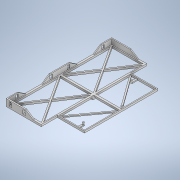
# Autodesk Inventor part: Wexterås-Hållare v2
Saved by Autodesk Inventor 2021 (Build 250183000, 183)
## iProperties
Created: 2024-12-11
Part Number: Wexterås-Hållare v2
Material: Generic
Document SubType Name: Modeling
Designer: 24ludrum
Density: 1 g/cm^3
Appearance: Default
Author: 24ludrum
Autodesk Inventor part; units mm, degrees
ref_plane "YZ Plane" through (0, 0, 0) normal (1, 0, 0) x (0, 1, 0)
ref_plane "XZ Plane" through (0, 0, 0) normal (0, 1, 0) x (-1, 0, 0)
ref_plane "XY Plane" through (0, 0, 0) normal (0, 0, 1) x (1, 0, 0)
sketch "Sketch1" plane through (0, 0, 0) normal (0, 1, 0) x (-1, 0, 0)
  line L0 (54, 0) -> (55.5, 0)
  line L1 (55.5, 0) -> (55.5, 82)
  line L2 (55.5, 82) -> (55.5, 83.5)
  line L3 (55.5, 83.5) -> (54, 83.5)
  line L4 (0, 83.5) -> (0, 82)
  line L5 (54, 82) -> (54, 80.5)
  line L6 (54, 82) -> (52.5, 82)
  line L7 (54, 0) -> (54, 1.5)
  line L8 (54, 1.5) -> (54, 80.5)
  line L9 (54, 0) -> (52.5, 0)
  line L10 (0, 1.5) -> (0, 0)
  line L11 (0, 0) -> (1.5, 0)
  line L12 (52.5, 82) -> (0, 1.5)
  line L13 (1.5, 0) -> (54, 80.5)
  line L14 (0, 83.5) -> (1.5, 83.5)
  line L15 (54, 83.5) -> (0, 83.5)
  line L16 (0, 82) -> (1.5, 82)
  line L17 (0, 82) -> (0, 80.5)
  line L18 (52.5, 82) -> (1.5, 82)
  line L19 (52.5, 0) -> (0, 80.5)
  line L20 (1.5, 82) -> (54, 1.5)
  line L21 (0, 0) -> (0, -0.1)
  line L22 (54, 0) -> (54, -0.1)
  line L23 (0, 0) -> (-43.1, 0)
  line L24 (0, 58) -> (0, 56.5)
  line L25 (0, 56.5) -> (0, 1.5)
  line L26 (-43.1, 1.5) -> (-43.1, 0)
  line L27 (-43.1, 58) -> (-43.1, 56.5)
  line L28 (-43.1, 56.5) -> (-43.1, 1.5)
  line L29 (0, 80.5) -> (0, 58)
  line L30 (1.5, 1.5) -> (52.5, 1.5)
  line L31 (52.5, 1.5) -> (52.5, 80.5)
  line L32 (0, 58) -> (-1.5, 58)
  line L33 (-43.1, 58) -> (-41.6, 58)
  line L34 (-1.5, 58) -> (-41.6, 58)
  line L35 (-41.6, 1.4999) -> (-1.3749, 1.4999)
  line L36 (-41.6, 1.4999) -> (-41.6, 56.5001)
  line L37 (52.5, 0) -> (1.5, 0)
  line L38 (55.5, 0) -> (55.5, -0.1)
  line L39 (52.5, 80.5) -> (1.5, 80.5)
  line L40 (1.5, 80.5) -> (1.5, 1.5)
  line L41 (-1.3749, 56.5001) -> (-41.6, 56.5001)
  line L42 (-1.3749, 56.5001) -> (-1.3749, 1.4999)
  line L43 (54, -0.1) -> (0, -0.1)
  line L44 (0, -0.1) -> (-43.1, -0.1)
  line L45 (-43.1, -0.1) -> (-43.1, 0)
  line L46 (54, -0.1) -> (55.5, -0.1)
  point P0 (27, 39.1)
  point P1 (51.5217, 1.5)
  point P2 (2.4783, 1.5)
  point P3 (25.7609, 41)
  point P4 (1.5, 3.8)
  point P5 (1.5, 78.2)
  point P6 (28.2391, 41)
  point P7 (52.5, 78.2)
  point P8 (52.5, 3.8)
  point P9 (27, 42.9)
  point P10 (2.4783, 80.5)
  point P11 (51.5217, 80.5)
  dimension "d0" = 82
  dimension "d1" = 54
  dimension "d2" = 82
  dimension "d3" = 1.5
  dimension "d4" = 1.5
  dimension "d5" = 1.5
  dimension "d6" = 1.5
  dimension "d8" = 1.5
  dimension "d9" = 1.5
  dimension "d10" = 1.5
  dimension "d12" = 1.5
  dimension "d13" = 1.5
  dimension "d14" = 1.5
  dimension "d15" = 1.5
  dimension "d16" = 1.5
  dimension "d17" = 0.1
  dimension "d18" = 0.1
  dimension "d19" = 43.1
  dimension "d20" = 58
  dimension "d21" = 1.5
  dimension "d22" = 1.5
  dimension "d23" = 55
  dimension "d24" = 1.5
  dimension "d25" = 1.5
  dimension "d26" = 51
  dimension "d27" = 54
  dimension "d28" = 51
  dimension "d31" = 40.2251
  dimension "d33" = 55.0001
  dimension "d34" = 1.5
  dimension "d35" = 0.1
  dimension "d37" = 1.5
  dimension "d38" = 1.4999
  dimension "d39" = 1.5
  constraints: 94 end point, 13 horizontal, 13 vertical, 9 perpendicular, 3 parallel, 2 point on line, 1 collinear
  measures "d0" distance of L0.start L5.start
  measures "d1" distance of L5.start L4.end
  measures "d2" distance of L0.end L1.end
  measures "d3" distance of L0.start L0.end
  measures "d4" distance of L1.end L2.end
  measures "d5" distance of L5.start L5.end
  measures "d6" distance of L5.start L6.end
  measures "d8" distance of L0.start L7.end
  measures "d9" distance of L0.start L9.end
  measures "d10" distance of L4.start L4.end
  measures "d12" distance of L10.end L11.end
  measures "d13" distance of L10.start L10.end
  measures "d14" distance of L4.start L14.end
  measures "d15" distance of L4.end L17.end
  measures "d16" distance of L4.end L16.end
  measures "d17" distance of L10.end L21.end
  measures "d18" distance of L0.start L22.end
  measures "d19" distance of L10.end L23.end
  measures "d20" distance of L23.end L27.start
  measures "d21" distance of L24.start L24.end
  measures "d22" distance of L27.start L27.end
  measures "d23" distance of L27.end L26.start
  measures "d24" distance of L24.start L32.end
  measures "d25" distance of L27.start L33.end
  measures "d26" distance of L30.start L30.end
  measures "d27" distance of L3.end L4.start
  measures "d28" distance of L18.start L16.end
  measures "d31" distance of L35.start L35.end
  measures "d33" distance of L35.start L36.end
  measures "d34" distance between parallel lines of L8 L31
  measures "d35" distance of L0.end L38.end
  measures "d37" distance between parallel lines of L39 L18
  measures "d38" distance between parallel lines of L34 L41
  measures "d39" distance between parallel lines of L28 L36
extrude "Extrusion1" add sketch "Sketch1" along normal blind 3 contours L7 L8 L5 L6 L18 L16 L4 L14 L15 L3 L2 L1 L0 | L9 L19 L30 L31 L20 L7 | L22 L43 L21 L11 L37 L9 | L20 L31 L13 L8 | L37 L13 L30 L19 | L13 L31 L39 L12 L6 L5 | L31 L30 L19 L13 L20 | L11 L10 L12 L40 L30 L13 | L44 L45 L23 L21 | L13 L20 L12 L39 L31 | L13 L19 L12 L20 | L13 L30 L40 L12 L19 | L23 L26 L28 L27 L33 L34 L32 L24 L25 L10 | L12 L39 L20 L18 | L12 L19 L40 L39 L20 | L25 L24 L29 L19 L40 L12 | L20 L39 L40 L19 L17 L16
sketch "Sketch3" plane through (-55.5, 0, 0) normal (-1, 0, 0) x (0, 0, 1)
  line L0 (3.8, 3) -> (78.2, 3) projected
  line L1 (11.2989, 4) -> (11.2989, 11)
  line L2 (11.2989, 4) -> (15.4989, 4)
  line L3 (15.4989, 11) -> (11.2989, 11)
  line L4 (15.4989, 11) -> (15.4989, 9.2)
  line L5 (15.4989, 9.2) -> (15.4989, 4)
  line L6 (15.4989, 9.2) -> (11.2989, 9.2)
  line L7 (58, 3) -> (0, 3) projected
  line L8 (11.2989, 11) -> (-0.7359, 2.9768)
  line L9 (15.4989, 11) -> (27.5338, 2.9768)
  line L10 (0, 3) -> (40.25, 3) construction
  line L11 (40.25, 3) -> (40.25, 23.325) construction
  line L12 (27.5338, 2.9768) -> (-0.7359, 2.9768)
  line L13 (70, 4) -> (70, 11)
  line L14 (70, 4) -> (65.8, 4)
  line L15 (65.8, 11) -> (70, 11)
  line L16 (65.8, 11) -> (65.8, 9.2)
  line L17 (65.8, 9.2) -> (65.8, 4)
  line L18 (65.8, 9.2) -> (70, 9.2)
  line L19 (65.8, 11) -> (53.8, 3)
  line L20 (56.5001, 0) -> (56.5001, 3) projected
  line L21 (83.5, 3) -> (58, 3) projected
  line L22 (56.5001, 3) -> (83.5, 3)
  line L23 (83.5, 3) -> (83.5, 11)
  line L24 (83.5, 11) -> (70, 11)
  line L25 (58, 3) -> (-0.1, 3) projected
  line L26 (55.3, 3) -> (58, 3)
  line L27 (55.3, 3) -> (83.5, 3)
  line L28 (53.8, 3) -> (55.3, 3)
  line L29 (0, 3) -> (-0.1, 3)
  line L30 (-0.1, 3) -> (0, 3) construction
  line L31 (-0.1, 3) -> (0, 3) construction
  line L32 (0, 3) -> (-0.1, 3) construction
  line L33 (83.5, 4) -> (15.5, 4) construction
  point P0 (0, 0)
  point P1 (80.5, 3)
  point P2 (53.8, 3)
  point P3 (27.4989, 3)
  point P4 (70, 11)
  point P5 (0, 3)
  point P6 (27.4989, 3)
  dimension "d45" = 4.2
  dimension "d47" = 5.2
  dimension "d49" = 1
  dimension "d50" = 7
  dimension "d52" = 33.69
  dimension "d55" = 1.8
  dimension "d56" = 33.69
  dimension "d57" = 40.25
  dimension "d93" = 8
  dimension "d94" = 13.5
  dimension "d95" = 33.69
  dimension "d96" = 4.2
  dimension "d97" = 4.2
  dimension "d98" = 1.8
  dimension "d99" = 12
  dimension "d100" = 5.2
  dimension "d101" = 7
  dimension "d102" = 4.2
  dimension "d103" = 1
  dimension "d104" = 90
  dimension "d112" = 68
  constraints: 56 end point, 7 horizontal, 4 point on line, 4 vertical, 1 parallel, 1 perpendicular, 1 symmetric about line, 1 other
  measures "d45" distance of L1.start L2.end
  measures "d47" distance of L4.end L2.end
  measures "d49" distance between parallel lines of L0 L2
  measures "d50" distance of L1.start L1.end
  measures "d52" angle of L7 L8
  measures "d55" distance between parallel lines of L6 L3
  measures "d56" angle of L0 L9
  measures "d57" distance of L7.end L10.end
  measures "d93" distance of L21.start L23.end
  measures "d94" distance of L23.end L24.end
  measures "d95" angle of L0 L19
  measures "d96" distance of L13.start L14.end
  measures "d97" distance of L18.start L18.end
  measures "d98" distance between parallel lines of L18 L15
  measures "d99" horizontal distance of L16.start L19.end
  measures "d100" distance of L18.start L14.end
  measures "d101" distance of L13.start L13.end
  measures "d102" distance of L16.start L13.end
  measures "d103" distance between parallel lines of L21 L14
  measures "d104" angle of L24 L13
  measures "d112" distance of L33.start L33.end
extrude "Extrusion2" add sketch "Sketch3" against normal blind 1.5 contours L19 L16 L17 L14 L13 L24 L23 L21 L0 | L15 L13 L18 L16 | L2 L5 L4 L9 L12 L8 L1 | L1 L3 L4 L6
extrude "Extrusion3" add sketch "Sketch1" along normal blind 3 contours L0 L38 L46 L22
mirror "Mirror1" about plane through (43.1, 0, -0.1) normal (0, 0, -1) of "Extrusion1", "Extrusion2"
sketch "Sketch4" plane through (-55.5, 0, 83.5) normal (0, 0, 1) x (1, 0, 0)
  line L0 (1.5, 0) -> (0, 0) projected
  line L1 (0, 0) -> (0, 11) projected
  line L2 (0, 0) -> (0, 11)
  line L3 (0, 11) -> (1.5, 11) projected
  line L4 (0, 11) -> (1.5, 11)
  line L5 (1.5, 11) -> (4.55, 11)
  line L6 (4.55, 11) -> (4.55, 4.6854)
  line L7 (4.55, 4.6854) -> (4.55, 0)
  line L8 (3.9783, 3) -> (53.0217, 3) projected
  line L9 (4.55, 3) -> (0, 3)
  line L10 (1.5, 3.4007) -> (1.5, 11) projected
  line L11 (1.5, 11) -> (1.5, 3)
  line L12 (4.55, 9) -> (8.75, 9)
  line L13 (4.55, 11) -> (8.75, 11)
  line L14 (8.75, 11) -> (8.75, 3)
  line L15 (8.75, 11) -> (26.55, 11)
  line L16 (26.55, 11) -> (26.55, 3)
  line L17 (26.55, 11) -> (30.75, 11)
  line L18 (26.55, 9) -> (32.35, 9)
  line L19 (30.75, 11) -> (30.75, 3)
  line L20 (30.75, 11) -> (43.0689, 3)
  line L21 (53.0217, 3) -> (3.9783, 3) projected
  point P0 (55.5, 0)
  point P1 (30.75, 9)
  dimension "d62" = 3.05
  dimension "d64" = 4.2
  dimension "d65" = 2
  dimension "d66" = 4.2
  dimension "d67" = 17.8
  dimension "d68" = 4.2
  dimension "d69" = 2
  dimension "d70" = 33
  constraints: 32 end point, 10 point on line, 5 horizontal, 4 perpendicular, 3 collinear, 2 vertical
  measures "d62" distance of L3.end L5.end
  measures "d64" distance of L12.start L12.end
  measures "d65" distance between parallel lines of L12 L13
  measures "d66" distance of L5.end L13.end
  measures "d67" distance of L13.end L15.end
  measures "d68" distance of L15.end L17.end
  measures "d69" distance between parallel lines of L18 L17
  measures "d70" angle of L20 L8
extrude "Extrusion4" add sketch "Sketch4" against normal blind 2 contours L11 L10 L5 L6 L7 L8 L9 | L13 L14 L12 L6 | L15 L16 L8 L14 | L17 L19 L18 L16 | L20 L8 L19
sketch "Sketch5" plane through (0, 0, -83.7) normal (0, 0, -1) x (-1, 0, 0)
  line L0 (55.5, 11) -> (54, 11) projected
  line L1 (54, 11) -> (24.75, 11) projected
  line L2 (55.5, 11) -> (24.75, 11)
  line L3 (24.75, 11) -> (12.4311, 3) projected
  line L4 (24.75, 11) -> (12.4311, 3)
  line L5 (12.4311, 3) -> (55.5, 3)
  line L6 (55.5, 3) -> (55.5, 11)
  point P0 (0, 0)
  constraints: 8 end point, 1 collinear, 1 horizontal, 1 parallel, 1 perpendicular
extrude "Extrusion5" add sketch "Sketch5" against normal blind 1.5
sketch "Sketch6" plane through (0, 0, 0) normal (0, -1, 0) x (1, 0, 0)
  line L0 (1.3749, 56.5001) -> (1.3749, 1.4999) construction
  line L1 (1.3749, 1.4999) -> (3.3749, 1.4999) construction
  line L2 (1.3749, 1.4999) -> (41.6, 1.4999) construction
  line L3 (1.3749, 1.4999) -> (1.3749, 4.4999) construction
  line L4 (1.3749, 4.4999) -> (3.3749, 4.4999) construction
  circle A0 centre (3.3749, 4.4999) radius 1.4 construction
  line L5 (3.3749, 5.8999) -> (1.3749, 5.8999) construction
  line L6 (3.3749, 3.0999) -> (3.3749, 1.4999) construction
  line L7 (3.3749, 3.0999) -> (3.3749, 1.4999)
  line L8 (3.3749, 5.8999) -> (1.3749, 5.8999)
  line L9 (1.3749, 5.8999) -> (1.3749, 1.4999)
  line L10 (3.3749, 1.4999) -> (1.3749, 1.4999)
  circle A1 centre (3.3749, 4.4999) radius 1.4
  line L11 (3.3749, 4.4999) -> (3.3749, 47.9999) construction
  line L12 (3.3749, 47.9999) -> (31.4749, 47.9999) construction
  circle A2 centre (31.4749, 47.9999) radius 1.4
  line L13 (32.8749, 47.9999) -> (32.8749, 56.5001)
  line L14 (30.0749, 47.9999) -> (30.0749, 56.5001)
  line L15 (41.6, 56.5001) -> (1.3749, 56.5001) projected
  line L16 (43.1, 58) -> (43.1, -58.2) construction
  line L17 (43.1, -0.1) -> (0, -0.1) construction
  line L18 (1.3749, -1.6999) -> (3.3749, -1.6999) construction
  line L19 (1.3749, -1.6999) -> (1.3749, -4.6999) construction
  line L20 (1.3749, -6.0999) -> (1.3749, -1.6999)
  line L21 (32.8749, -56.7001) -> (30.0749, -56.7001)
  line L22 (41.6, -56.7001) -> (1.3749, -56.7001) projected
  line L23 (32.8749, 56.5001) -> (30.0749, 56.5001)
  line L24 (1.3749, -1.6999) -> (41.6, -1.6999) construction
  line L25 (41.6, -1.6999) -> (38.4273, -1.6999) construction
  line L26 (41.6, -1.6999) -> (41.6, -3.8999) construction
  line L27 (41.6, -1.6999) -> (41.6, -56.7001) construction
  line L28 (41.6, -1.6999) -> (41.6, -4.6999)
  line L29 (41.6, -1.6999) -> (39.6, -1.6999)
  line L30 (39.6, -1.6999) -> (39.6, -4.6999)
  circle A3 centre (39.6, -4.6999) radius 1.4
  line L31 (39.6, -4.6999) -> (11.5, -4.6999) construction
  line L32 (11.5, -4.6999) -> (11.5, -48.1999) construction
  circle A4 centre (11.5, -48.1999) radius 1.4
  line L33 (10.1, -48.1999) -> (10.1, -56.7001)
  line L34 (12.9, -48.1999) -> (12.9, -56.7001)
  line L35 (12.9, -56.7001) -> (10.1, -56.7001)
  line L36 (41.6, -4.6999) -> (39.6, -4.6999)
  line L37 (41.6, -1.6999) -> (41.6, -56.7001) projected
  line L38 (39.6, -1.6999) -> (39.6, -4.6999)
  line L39 (1.3749, -1.6999) -> (41.6, -1.6999) projected
  point P0 (0, 0)
  point P1 (41, -4.6999)
  point P2 (39.6, -3.2999)
  dimension "d75" = 2
  dimension "d76" = 3
  dimension "d77" = 2.8
  dimension "d78" = 43.5
  dimension "d79" = 28.1
  dimension "d80" = 2.8
  dimension "d115" = 3
  dimension "d116" = 2
  dimension "d117" = 2.8
  dimension "d118" = 28.1
  dimension "d119" = 43.5
  dimension "d120" = 2.8
  constraints: 62 end point, 9 point on line, 8 perpendicular, 6 point on circle, 6 symmetric about line, 6 vertical, 5 centre point, 4 coincident, 4 collinear, 4 horizontal, 1 concentric, 1 midpoint, 1 parallel
  measures "d75" distance of L1.end L0.end
  measures "d76" distance of L3.end L0.end
  measures "d77" diameter of A0
  measures "d78" distance of L11.start L11.end
  measures "d79" distance of L11.end L12.end
  measures "d80" diameter of A2
  measures "d115" distance of L28.end L24.end
  measures "d116" distance of L24.end L29.end
  measures "d117" diameter of A3
  measures "d118" distance of L31.start L31.end
  measures "d119" distance of L31.end L32.end
  measures "d120" diameter of A4
extrude "Extrusion6" add sketch "Sketch6" against normal blind 1.5 contours L7 L10 L9 L8 A1 | A2 L14 L15 L13 | L22 L33 A4 L34 | L28 L36 A3 L30 L29
extrude "Extrusion7" add sketch "Sketch6" against normal blind 4.2 contours A1 | A2 | A4 | L36 L30 A3 | A3 L30 L36
sketch "Sketch7" plane through (0, 0, 0) normal (0, -1, 0) x (1, 0, 0)
  line L0 (41.6, 1.4999) -> (41.6, 2.9999)
  line L1 (41.6, 1.4999) -> (40.1, 1.4999)
  line L2 (3.3749, 1.4999) -> (41.6, 1.4999) projected
  line L3 (30.0749, 56.5001) -> (1.3749, 56.5001) projected
  line L4 (1.3749, 56.5001) -> (2.8749, 56.5001)
  line L5 (1.3749, 56.5001) -> (1.3749, 55.0001)
  line L6 (1.3749, 56.5001) -> (1.3749, 5.8999) projected
  line L7 (2.8749, 56.5001) -> (41.6, 2.9999)
  line L8 (40.1, 1.4999) -> (1.3749, 55.0001)
  line L9 (43.1, 58) -> (43.1, -58.2) construction
  line L10 (43.1, -0.1) -> (0, -0.1) construction
  line L11 (41.6, -1.6999) -> (41.6, -3.1999)
  line L12 (41.6, -1.6999) -> (40.1, -1.6999)
  line L13 (30.0749, -56.7001) -> (1.3749, -56.7001)
  line L14 (1.3749, -56.7001) -> (1.3749, -55.2001)
  line L15 (2.8749, -56.7001) -> (41.6, -3.1999)
  line L16 (40.1, -1.6999) -> (1.3749, -55.2001)
  point P0 (0, 0)
  dimension "d85" = 1.5
  dimension "d86" = 1.5
  dimension "d87" = 1.5
  dimension "d88" = 1.5
  constraints: 26 end point, 7 symmetric about line, 4 point on line, 1 horizontal, 1 midpoint, 1 vertical
  measures "d85" distance of L0.start L0.end
  measures "d86" distance of L0.start L1.end
  measures "d87" distance of L4.end L3.end
  measures "d88" distance of L3.end L5.end
extrude "Extrusion8" add sketch "Sketch7" against normal blind 1.5
extrude "Extrusion9" add sketch "Sketch3" against normal blind 1.5 contours L19 L16 L17 L14 L13 L24 L23 L21 L0
sketch "Sketch13" plane through (-55.5, 0, -0.2) normal (0, 0, 1) x (1, 0, 0)
  line L0 (0, 11) -> (0, 3.4007) projected
  line L1 (1.5, 0) -> (1.5, 2.9768) projected
  line L2 (0, 3.4007) -> (1.5, 3.4007)
  line L3 (1.5, 3.4007) -> (1.5, 0)
  line L4 (1.5, 0) -> (0, 0)
  line L5 (0, 0) -> (0, 3.4007)
  point P0 (55.5, 0)
  point P1 (1.5, 3)
  constraints: 8 end point, 2 parallel, 1 horizontal, 1 perpendicular
extrude "Extrusion11" add sketch "Sketch13" along normal blind 0.1
sketch "Sketch14" plane through (-55.5, 11, 11.2989) normal (-1, 0, 0) x (0, 0, 1)
  line L0 (-11.3989, -7.5993) -> (-22.7979, 0) projected
  line L1 (0, 0) -> (4.2, 0) projected
  line L2 (-22.7979, 0) -> (0, 0)
  line L3 (0, 0) -> (-11.3989, -7.5993)
  line L4 (-11.3989, -7.5993) -> (-22.7979, 0)
  point P0 (-11.2989, -11)
  constraints: 6 end point, 1 horizontal
extrude "Extrusion12" add sketch "Sketch14" against normal blind 1.5
equation "\"d56\" = d52"
body "Solid1"
